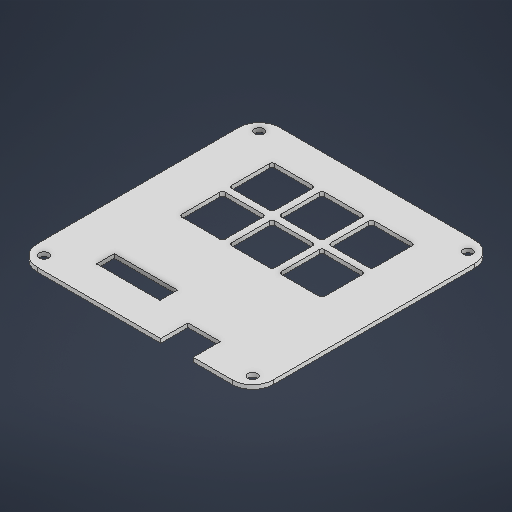
# Autodesk Inventor part: case top
Saved by Autodesk Inventor 2026 (Build 300175050, 175E)
## iProperties
Created: 2025-06-25
Part Number: case top
Material: Generic
Document SubType Name: Modeling
Designer: shlinke
Density: 1 g/cm^3
Appearance: Default
Autodesk Inventor part; units mm, degrees
ref_plane "YZ Plane" through (0, 0, 0) normal (1, 0, 0) x (0, 1, 0)
ref_plane "XZ Plane" through (0, 0, 0) normal (0, 1, 0) x (-1, 0, 0)
ref_plane "XY Plane" through (0, 0, 0) normal (0, 0, 1) x (1, 0, 0)
sketch "Sketch3" plane through (0, 0, 0) normal (0, 1, 0) x (-1, 0, 0)
  line L0 (-25.241, 1.984) -> (-11.271, 1.984)
  line L1 (-25.241, -13.891) -> (-11.271, -13.891)
  line L2 (-26.1935, 1.0315) -> (-26.1935, -12.9385)
  line L3 (-10.3185, 1.0315) -> (-10.3185, -12.9385)
  arc A0 (-25.241, 1.984) -> (-26.1935, 1.0315) centre (-25.241, 1.0315) ccw
  arc A1 (-10.3185, 1.0315) -> (-11.271, 1.984) centre (-11.271, 1.0315) ccw
  arc A2 (-26.1935, -12.9385) -> (-25.241, -13.891) centre (-25.241, -12.9385) ccw
  arc A3 (-11.271, -13.891) -> (-10.3185, -12.9385) centre (-11.271, -12.9385) ccw
  line L4 (-6.985, 1.984) -> (6.985, 1.984)
  line L5 (-6.985, -13.891) -> (6.985, -13.891)
  line L6 (-7.9375, 1.0315) -> (-7.9375, -12.9385)
  line L7 (7.9375, 1.0315) -> (7.9375, -12.9385)
  arc A4 (-6.985, 1.984) -> (-7.9375, 1.0315) centre (-6.985, 1.0315) ccw
  arc A5 (7.9375, 1.0315) -> (6.985, 1.984) centre (6.985, 1.0315) ccw
  arc A6 (-7.9375, -12.9385) -> (-6.985, -13.891) centre (-6.985, -12.9385) ccw
  arc A7 (6.985, -13.891) -> (7.9375, -12.9385) centre (6.985, -12.9385) ccw
  line L8 (11.271, 1.984) -> (25.241, 1.984)
  line L9 (11.271, -13.891) -> (25.241, -13.891)
  line L10 (10.3185, 1.0315) -> (10.3185, -12.9385)
  line L11 (26.1935, 1.0315) -> (26.1935, -12.9385)
  arc A8 (11.271, 1.984) -> (10.3185, 1.0315) centre (11.271, 1.0315) ccw
  arc A9 (26.1935, 1.0315) -> (25.241, 1.984) centre (25.241, 1.0315) ccw
  arc A10 (10.3185, -12.9385) -> (11.271, -13.891) centre (11.271, -12.9385) ccw
  arc A11 (25.241, -13.891) -> (26.1935, -12.9385) centre (25.241, -12.9385) ccw
  line L12 (-25.241, -16.272) -> (-11.271, -16.272)
  line L13 (-25.241, -32.147) -> (-11.271, -32.147)
  line L14 (-26.1935, -17.2245) -> (-26.1935, -31.1945)
  line L15 (-10.3185, -17.2245) -> (-10.3185, -31.1945)
  arc A12 (-25.241, -16.272) -> (-26.1935, -17.2245) centre (-25.241, -17.2245) ccw
  arc A13 (-10.3185, -17.2245) -> (-11.271, -16.272) centre (-11.271, -17.2245) ccw
  arc A14 (-26.1935, -31.1945) -> (-25.241, -32.147) centre (-25.241, -31.1945) ccw
  arc A15 (-11.271, -32.147) -> (-10.3185, -31.1945) centre (-11.271, -31.1945) ccw
  line L16 (-6.985, -16.272) -> (6.985, -16.272)
  line L17 (-6.985, -32.147) -> (6.985, -32.147)
  line L18 (-7.9375, -17.2245) -> (-7.9375, -31.1945)
  line L19 (7.9375, -17.2245) -> (7.9375, -31.1945)
  arc A16 (-6.985, -16.272) -> (-7.9375, -17.2245) centre (-6.985, -17.2245) ccw
  arc A17 (7.9375, -17.2245) -> (6.985, -16.272) centre (6.985, -17.2245) ccw
  arc A18 (-7.9375, -31.1945) -> (-6.985, -32.147) centre (-6.985, -31.1945) ccw
  arc A19 (6.985, -32.147) -> (7.9375, -31.1945) centre (6.985, -31.1945) ccw
  line L20 (11.271, -16.272) -> (25.241, -16.272)
  line L21 (11.271, -32.147) -> (25.241, -32.147)
  line L22 (10.3185, -17.2245) -> (10.3185, -31.1945)
  line L23 (26.1935, -17.2245) -> (26.1935, -31.1945)
  arc A20 (11.271, -16.272) -> (10.3185, -17.2245) centre (11.271, -17.2245) ccw
  arc A21 (26.1935, -17.2245) -> (25.241, -16.272) centre (25.241, -17.2245) ccw
  arc A22 (10.3185, -31.1945) -> (11.271, -32.147) centre (11.271, -31.1945) ccw
  arc A23 (25.241, -32.147) -> (26.1935, -31.1945) centre (25.241, -31.1945) ccw
  line L24 (-33.3375, -34.528) -> (33.3375, -34.528)
  line L25 (-33.3375, 34.528) -> (33.3375, 34.528)
  line L26 (-33.3375, -34.528) -> (-33.3375, 34.528)
  line L27 (33.3375, -34.528) -> (33.3375, 34.528)
  line L28 (-33.3375, 34.528) -> (-22.4409, 34.528) construction
  line L29 (-22.4409, 34.528) -> (-3.9497, 34.528)
  line L30 (-43.3375, -44.528) -> (43.3375, -44.528)
  line L31 (43.3375, -44.528) -> (43.3375, 44.528)
  line L32 (43.3375, 44.528) -> (-43.3375, 44.528)
  line L33 (-43.3375, 44.528) -> (-43.3375, -44.528)
  circle A24 centre (-38.3375, -39.528) radius 1.7
  circle A25 centre (38.3375, -39.528) radius 1.7
  circle A26 centre (-38.3375, 39.528) radius 1.7
  circle A27 centre (38.3375, 39.528) radius 1.7
  line L34 (-22.4409, 34.528) -> (-3.9409, 34.528)
  line L35 (-21.4315, 34.528) -> (-9.5255, 34.528)
  line L36 (-9.5255, 34.528) -> (-9.5255, 48.1303)
  line L37 (-9.5255, 48.1303) -> (-21.4315, 48.1303)
  line L38 (-21.4315, 48.1303) -> (-21.4315, 34.528)
  line L39 (2.7875, 26.028) -> (26.0375, 26.028)
  line L40 (26.0375, 26.028) -> (26.0375, 32.528)
  line L41 (26.0375, 32.528) -> (2.7875, 32.528)
  line L42 (2.7875, 32.528) -> (2.7875, 26.028)
  point P0 (0, 0)
  point P1 (-10.3185, -5.9535)
  point P2 (0, 0)
  point P3 (-21.4315, 44.528)
  point P4 (-9.5255, 44.528)
  point P5 (-9.5255, 34.528)
  dimension "d13" = 2.381
  dimension "d14" = 7.144
  dimension "d15" = 66.675
  dimension "d16" = 69.056
  dimension "d17" = 7.144
  dimension "d18" = 13.97
  dimension "d19" = 13.97
  dimension "d20" = 2.381
  dimension "d21" = 13.97
  dimension "d22" = 13.97
  dimension "d23" = 13.97
  dimension "d24" = 2.381
  dimension "d25" = 2.381
  dimension "d46" = 10
  dimension "d47" = 10
  dimension "d48" = 3.4
  dimension "d49" = 3.4
  dimension "d50" = 3.4
  dimension "d51" = 3.4
  dimension "d52" = 5
  dimension "d53" = 5
  dimension "d54" = 5
  dimension "d55" = 5
  dimension "d56" = 5
  dimension "d57" = 5
  dimension "d58" = 5
  dimension "d59" = 5
  dimension "d62" = 11.906
  dimension "d66" = 23.25
  dimension "d67" = 6.5
  dimension "d72" = 7.3
  dimension "d73" = 2
  dimension "d74" = 10
  constraints: 86 end point, 66 tangent, 48 point on circle, 28 centre point, 23 equal radius, 20 parallel, 11 perpendicular, 6 horizontal, 1 coincident, 1 collinear, 1 midpoint, 1 point on line
  measures "d13" distance between parallel lines of L24 L13
  measures "d14" distance between parallel lines of L26 L14
  measures "d15" distance of L24.start L24.end
  measures "d16" distance of L24.start L26.end
  measures "d17" distance between parallel lines of L27 L23
  measures "d18" distance of L23.start L23.end
  measures "d19" distance of L21.start L21.end
  measures "d20" distance between parallel lines of L5 L16
  measures "d21" distance of L3.start L3.end
  measures "d22" distance of L1.start L1.end
  measures "d23" distance of L5.start L5.end
  measures "d24" distance between parallel lines of L10 L7
  measures "d25" distance from line of point (-10.318, -5.953) L6
  measures "d46" distance between parallel lines of L31 L27
  measures "d47" distance between parallel lines of L32 L25
  measures "d48" diameter of A24
  measures "d49" diameter of A25
  measures "d50" diameter of A26
  measures "d51" diameter of A27
  measures "d52" distance from line of L32 A26.centre
  measures "d53" distance from line of L33 A26.centre
  measures "d54" distance from line of L32 A27.centre
  measures "d55" distance from line of L31 A27.centre
  measures "d56" distance from line of L31 A25.centre
  measures "d57" distance from line of L30 A25.centre
  measures "d58" distance from line of L30 A24.centre
  measures "d59" distance from line of L33 A24.centre
  measures "d62" distance of L37.end L36.end
  measures "d66" distance of L41.end L40.end
  measures "d67" distance of L39.end L40.end
  measures "d72" distance between parallel lines of L27 L40
  measures "d73" distance between parallel lines of L25 L41
  measures "d74" distance between parallel lines of L33 L26
extrude "Extrusion4" add sketch "Sketch3" along normal blind 1.5 contours L26 L25 L27 L24 | L24 L27 L25 L36 L32 L31 L30 L33 L38 L26
fillet "Fillet4" radius 7.5 4 edges at (-43.3375, 0.75, -44.528) (-43.3375, 0.75, 44.528) (43.3375, 0.75, -44.528) (43.3375, 0.75, 44.528)
body "Solid4"
